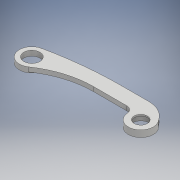
# Autodesk Inventor part: Arm 13X - parallel linkage
Saved by Autodesk Inventor 2017 (Build 210142000, 142)
## iProperties
Created: 2016-03-31
Part Number: Arm 13X - parallel linkage
Material: Generic
Document SubType Name: Modeling
Designer: alist
Density: 1 g/cm^3
Appearance: Default
Author: alist
## iProperties of the stored document Arm - parallel linkage_3DPrint.ipt
Created: 2017-01-15
Part Number: Arm - parallel linkage_3DPrint
Material: Generic
Document SubType Name: Modeling
Designer: Alistair
Density: 1 g/cm^3
Appearance: Default
Author: Alistair
Autodesk Inventor part; units mm, degrees
ref_plane "YZ Plane" through (0, 0, 0) normal (1, 0, 0) x (0, 1, 0)
ref_plane "XZ Plane" through (0, 0, 0) normal (0, 1, 0) x (-1, 0, 0)
ref_plane "XY Plane" through (0, 0, 0) normal (0, 0, 1) x (1, 0, 0)
sketch "Sketch1" plane through (0, 0, 0) normal (0, 0, 1) x (1, 0, 0)
  circle A0 centre (-74.2, 0) radius 11
  circle A1 centre (74.2, 0) radius 11
  arc A2 (-77.7059, 16.6346) -> (-64.5678, -14.0079) centre (-74.2, 0) ccw
  arc A3 (57.2488, -1.2867) -> (88.0183, 9.9023) centre (74.2, 0) ccw
  line L0 (-103.108, 0) -> (101.0811, 0)
  line L1 (48.335, 6.976) -> (2.9837, 6.976)
  arc A4 (2.9837, 6.976) -> (-64.5678, -14.0079) centre (2.9837, -112.247) ccw
  arc A5 (57.2488, -1.2867) -> (48.335, 6.976) centre (48.335, -1.9634) ccw
  line L2 (88.0183, 9.9023) -> (85.9436, 12.7975)
  line L3 (21.5061, 26.976) -> (58.34, 26.976)
  arc A6 (85.9436, 12.7975) -> (58.34, 26.976) centre (58.34, -6.9833) ccw
  arc A7 (21.5061, 26.976) -> (-77.7059, 16.6346) centre (21.5061, -454.096) ccw
  point P0 (0, 0)
  dimension "d0" = 22
  dimension "d1" = 22
  dimension "d2" = 148.4
  dimension "d3" = 74.2
  dimension "d4" = 6
  dimension "d5" = 6
  dimension "d12" = 20
  constraints: 12 point on circle, 9 tangent, 8 centre point, 8 end point, 3 horizontal, 3 point on line
  measures "d0" diameter of A0
  measures "d1" diameter of A1
  measures "d2" distance of A1.centre A0.centre
  measures "d3" distance of A1.centre point (0, 0)
  measures "d4" radial gap between concentric circles of A0 A2
  measures "d5" radial gap between concentric circles of A1 A3
  measures "d12" distance between parallel lines of L3 L1
extrude "Extrusion1" add sketch "Sketch1" along normal blind 6 contours L0 A4 A2 A0 | A0 L0 A2 A7 L3 A6 L2 A3 A1 A5 L1 A4 | L0 A1 A3 A5
sketch "Sketch2" plane through (0, 0, 6) normal (0, 0, 1) x (1, 0, 0)
  circle A0 centre (-74.2, 0) radius 11 projected
  circle A1 centre (-74.2, 0) radius 17
  circle A2 centre (74.2, 0) radius 11 projected
  circle A3 centre (74.2, 0) radius 17
  point P0 (0, 0)
  constraints: 2 centre point, 2 coincident
extrude "Extrusion2" add sketch "Sketch2" against normal blind 9
fillet "Fillet1" [suppressed]
sketch "Sketch3" plane through (0, 0, 6) normal (0, 0, 1) x (1, 0, 0)
  circle A0 centre (74.2, 0) radius 11 projected
  circle A1 centre (74.2, 0) radius 9
  point P0 (0, 0)
  dimension "d32" = 18
  constraints: 1 centre point, 1 coincident
  measures "d32" diameter of A1
extrude "Extrusion3" add sketch "Sketch3" against normal blind 2
sketch "Sketch5" plane through (-74.2, 0, -3) normal (0, 0, -1) x (-1, 0, 0)
  circle A0 centre (0, 0) radius 11 projected
  circle A1 centre (0, 0) radius 17 projected
  point P0 (-74.2, 0)
extrude "Extrusion5" cut sketch "Sketch5" against normal blind 2
equation "\"d3\" = 0.5 * d2"
body "Solid1"
